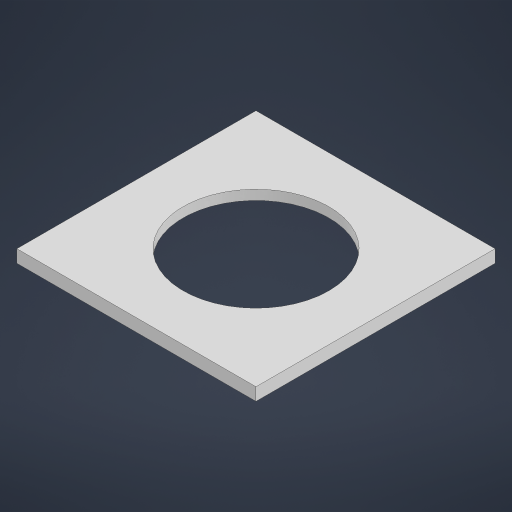
# Autodesk Inventor part: Silicone_Spreader
Saved by Autodesk Inventor 2024.1 (Build 281209000, 209)
## iProperties
Created: 2024-08-16
Part Number: Silicone_Spreader
Material: Generic
Document SubType Name: Modeling
Designer: Tim Jäger
Density: 1 g/cm^3
Appearance: Default
Author: Tim Jäger
Autodesk Inventor part; units mm, degrees
ref_plane "YZ Plane" through (0, 0, 0) normal (1, 0, 0) x (0, 1, 0)
ref_plane "XZ Plane" through (0, 0, 0) normal (0, 1, 0) x (-1, 0, 0)
ref_plane "XY Plane" through (0, 0, 0) normal (0, 0, 1) x (1, 0, 0)
sketch "Sketch1" plane through (0, 0, 0) normal (0, 1, 0) x (-1, 0, 0)
  line L0 (-9.3, 9.3) -> (9.3, 9.3)
  line L1 (9.3, 9.3) -> (9.3, -9.3)
  line L2 (9.3, -9.3) -> (-9.3, -9.3)
  line L3 (-9.3, -9.3) -> (-9.3, 9.3)
  line L4 (-9.3, 9.3) -> (9.3, -9.3) construction
  line L5 (9.3, 9.3) -> (-9.3, -9.3) construction
  line L6 (-12.3, -12.3) -> (12.3, -12.3)
  line L7 (12.3, -12.3) -> (12.3, 12.3)
  line L8 (12.3, 12.3) -> (-12.3, 12.3)
  line L9 (-12.3, 12.3) -> (-12.3, -12.3)
  point P0 (0, 0)
  dimension "d0" = 18.6
  dimension "d1" = 18.6
  dimension "d2" = 3
  constraints: 20 end point, 4 parallel, 2 midpoint, 2 perpendicular, 1 horizontal, 3 other
  measures "d0" distance of L1.end L2.end
  measures "d1" distance of L0.end L1.end
  measures "d2" distance between parallel lines of L2 L6
extrude "Extrusion1" add sketch "Sketch1" along normal blind 0.3
sketch "Sketch2" plane through (0, 0.3, 0) normal (0, 1, 0) x (1, 0, 0)
  line L0 (-12.3, 12.3) -> (-12.3, -12.3) projected
  line L1 (-12.3, -12.3) -> (12.3, -12.3) projected
  line L2 (12.3, -12.3) -> (12.3, 12.3) projected
  line L3 (12.3, 12.3) -> (-12.3, 12.3) projected
  line L4 (9.3, -9.3) -> (-9.3, -9.3) construction
  line L5 (-9.3, -9.3) -> (-9.3, 9.3) construction
  line L6 (-9.3, 9.3) -> (9.3, 9.3) construction
  line L7 (9.3, 9.3) -> (9.3, -9.3) construction
  circle A0 centre (0, 0) radius 7.5
  dimension "d5" = 15
  constraints: 1 centre point, 1 coincident
  measures "d5" diameter of A0
extrude "Extrusion2" add sketch "Sketch2" along normal blind 1
body "Solid1"
